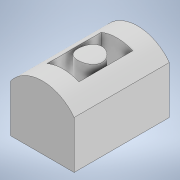
# Autodesk Inventor part: complex extrusion 1 5.7.20
Saved by Autodesk Inventor 2021 (Build 250183000, 183)
## iProperties
Created: 2020-05-07
Part Number: complex extrusion 1 5.7.20
Material: Generic
Document SubType Name: Modeling
Designer: david
Density: 1 g/cm^3
Appearance: Default
Author: david
Autodesk Inventor part; units mm, degrees
ref_plane "YZ Plane" through (0, 0, 0) normal (1, 0, 0) x (0, 1, 0)
ref_plane "XZ Plane" through (0, 0, 0) normal (0, 1, 0) x (-1, 0, 0)
ref_plane "XY Plane" through (0, 0, 0) normal (0, 0, 1) x (1, 0, 0)
sketch "Sketch1" plane through (0, 0, 0) normal (0, 1, 0) x (-1, 0, 0)
  line L0 (169.4818, -66.9774) -> (67.8818, -66.9774)
  line L1 (67.8818, -66.9774) -> (67.8818, -219.3774)
  line L2 (67.8818, -219.3774) -> (169.4818, -219.3774)
  line L3 (169.4818, -219.3774) -> (169.4818, -66.9774)
  point P0 (0, 0)
  dimension "d0" = 152.4
  dimension "d1" = 101.6
  constraints: 8 end point, 2 parallel, 1 horizontal, 1 perpendicular
  measures "d0" distance of L0.end L1.end
  measures "d1" distance of L0.start L0.end
extrude "Extrusion1" add sketch "Sketch1" along normal blind 101.6
sketch "Sketch2" plane through (0, 101.6, 0) normal (0, 1, 0) x (1, 0, 0)
  line L0 (-144.0818, 99.9974) -> (-93.2818, 99.9974)
  line L1 (-93.2818, 99.9974) -> (-93.2818, 186.3574)
  line L2 (-93.2818, 186.3574) -> (-144.0818, 186.3574)
  line L3 (-144.0818, 186.3574) -> (-144.0818, 99.9974)
  circle A0 centre (-118.6818, 143.1774) radius 19.2808
  line L4 (-67.8818, 219.3774) -> (-169.4818, 219.3774) projected
  line L5 (-169.4818, 66.9774) -> (-67.8818, 66.9774) projected
  line L6 (-169.4818, 219.3774) -> (-169.4818, 66.9774) projected
  line L7 (-67.8818, 66.9774) -> (-67.8818, 219.3774) projected
  point P0 (0, 0)
  dimension "d4" = 33.02
  dimension "d5" = 33.02
  dimension "d6" = 76.2
  dimension "d7" = 50.8
  dimension "d8" = 25.4
  dimension "d9" = 25.4
  constraints: 8 end point, 2 parallel, 1 centre point, 1 horizontal, 1 perpendicular
  measures "d4" distance between parallel lines of L4 L2
  measures "d5" distance between parallel lines of L0 L5
  measures "d6" distance from line of L4 A0.centre
  measures "d7" distance from line of L6 A0.centre
  measures "d8" distance between parallel lines of L6 L3
  measures "d9" distance between parallel lines of L7 L1
extrude "Extrusion2" cut sketch "Sketch2" against normal blind 63.5 contours L3 L2 L1 L0
sketch "Sketch3" plane through (-169.4818, 0, -66.9774) normal (0, 0, 1) x (1, 0, 0)
  line L0 (101.6, 0) -> (0, 0) projected
  arc A0 (101.6, 0) -> (0, 0) centre (50.8, 38.1) ccw
  line L1 (76.2, 101.6) -> (25.4, 101.6) projected
  point P0 (169.4818, 0)
  constraints: 2 point on circle, 1 centre point, 1 tangent
extrude "Extrusion3" cut sketch "Sketch3" against normal up to surface (152.4 mm away) keep common part
body "Solid1"
